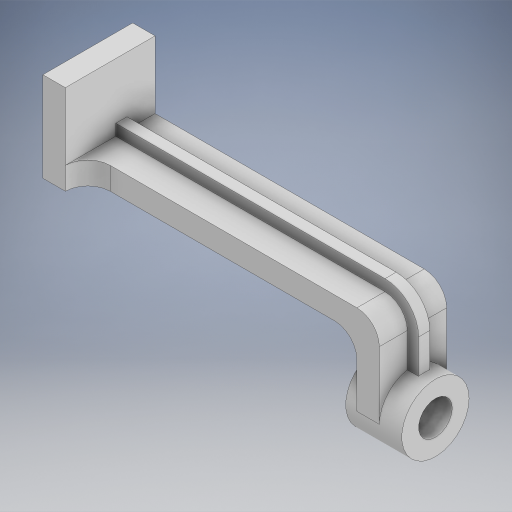
# Autodesk Inventor part: CE-1.4.2
Saved by Autodesk Inventor 2024 (Build 280153000, 153)
## iProperties
Created: 2024-01-25
Part Number: CE-1.4.2
Material: Generic
Document SubType Name: Modeling
Designer: Alex
Density: 1 g/cm^3
Appearance: Default
Author: Alex
Autodesk Inventor part; units mm, degrees
ref_plane "YZ Plane" through (0, 0, 0) normal (1, 0, 0) x (0, 1, 0)
ref_plane "XZ Plane" through (0, 0, 0) normal (0, 1, 0) x (-1, 0, 0)
ref_plane "XY Plane" through (0, 0, 0) normal (0, 0, 1) x (1, 0, 0)
sketch "Sketch1" plane through (0, 0, 0) normal (0, 0, 1) x (1, 0, 0)
  line L0 (0, 0) -> (12.7, 0)
  line L1 (12.7, 0) -> (12.7, 50.8)
  line L2 (12.7, 50.8) -> (0, 50.8)
  line L3 (0, 50.8) -> (0, 0)
  line L4 (12.7, 0) -> (152.4, 0)
  line L5 (165.1, 12.7) -> (12.7, 12.7)
  line L6 (12.7, 12.7) -> (12.7, 0) construction
  line L7 (165.1, 12.7) -> (165.1, 12.7)
  line L8 (177.8, 0) -> (177.8, -38.1)
  line L9 (177.8, -38.1) -> (165.1, -38.1)
  line L10 (165.1, -38.1) -> (165.1, -12.7)
  arc A0 (165.1, -12.7) -> (152.4, 0) centre (152.4, -12.7) ccw
  arc A1 (177.8, 0) -> (165.1, 12.7) centre (165.1, 0) ccw
  point P0 (177.8, 12.7)
  point P1 (12.7, 12.7)
  dimension "d0" = 50.8
  dimension "d1" = 12.7
  dimension "d2" = 50.8
  dimension "d3" = 12.7
  dimension "d4" = 177.8
  dimension "d5" = 12.7
  dimension "d6" = 12.7
  constraints: 22 end point, 5 parallel, 4 point on circle, 4 tangent, 3 horizontal, 2 centre point, 2 perpendicular, 2 point on line, 1 equal radius
  measures "d0" distance of L2.end L0.start
  measures "d1" distance of L0.start L0.end
  measures "d2" distance of point (177.8, 12.7) L8.end
  measures "d3" distance of L8.end L9.end
  measures "d4" distance between parallel lines of L3 L8
  measures "d5" distance between parallel lines of L5 L4
  measures "d6" radius of A0
extrude "Extrusion1" add sketch "Sketch1" along normal blind 50.8 contours L3 L2 L1 L0
extrude "Extrusion2" add sketch "Sketch1" along normal blind 38.1 contours L1 L5 A1 L8 L9 L10 A0 L4
fillet "Fillet1" radius 12.7 1 edges at (12.7, 6.35, 38.1)
sketch "Sketch2" plane through (177.8, -38.1, 0) normal (1, 0, 0) x (0, 0, -1)
  line L0 (0, 0) -> (-38.1, 0) projected
  circle A0 centre (-19.05, 0) radius 19.05
  point P0 (0, 38.1)
  constraints: 1 horizontal alignment, 1 midpoint, 2 other
extrude "Extrusion3" add sketch "Sketch2" along normal blind 12.7 and the other way blind 19.05
sketch "Sketch4" plane through (190.5, -38.1, 19.05) normal (1, 0, 0) x (0, 0, -1)
  circle A0 centre (0, 0) radius 19.05 projected
  point P0 (19.05, 38.1)
  constraints: 1 coincident
hole "Hole1" at (190.5, -38.1, 19.05) direction (-1, 0, 0) diameter 19.05 depth 31.75 tip angle 118
ref_plane "Work Plane1" through (0, 0, 19.05) normal (0, 0, 1) x (1, 0, 0)
sketch "Sketch5" plane through (0, 0, 19.05) normal (0, 0, 1) x (1, 0, 0)
  line L0 (165.1, 12.7) -> (25.4, 12.7) construction
  arc A0 (177.8, 0) -> (165.1, 12.7) centre (165.1, 0) ccw construction
  line L1 (177.8, -38.1) -> (177.8, 0) construction
  line L2 (25.4, 12.7) -> (12.7, 12.7) construction
  line L3 (12.7, 19.05) -> (25.4, 19.05)
  line L4 (25.4, 19.05) -> (165.1, 19.05)
  arc A1 (184.15, 0) -> (165.1, 19.05) centre (165.1, 0) ccw
  line L5 (184.15, 0) -> (184.15, -19.05)
  line L6 (158.75, -19.05) -> (190.5, -19.05) construction
  point P0 (0, 0)
  dimension "d23" = 6.35
  dimension "d24" = 152.4
  dimension "d25" = 165.1
  constraints: 6 end point, 2 point on circle, 1 centre point, 1 parallel, 1 point on line, 1 tangent, 2 other
  measures "d23" distance between parallel lines of L0 L4
  measures "d24" distance from line of L3.end L1
  measures "d25" distance from line of L3.start L1
extrude "Rib1" add sketch "Sketch5" along normal mid plane 6.35 rib yes fills toward (19.05, 19) open curves L3 L4 A1 L5
body "Solid1"
